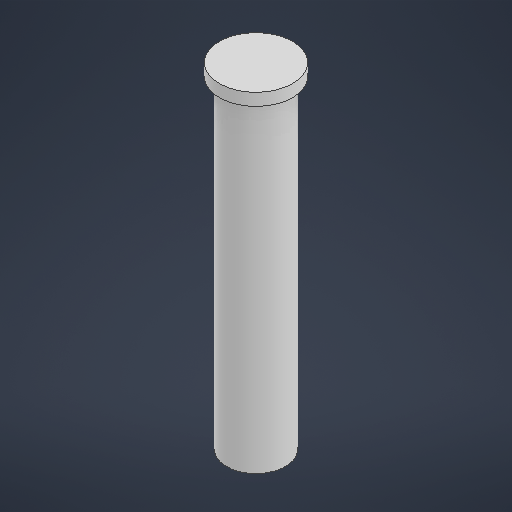
# Autodesk Inventor part: Press_Head
Saved by Autodesk Inventor 2026.1 (Build 301233020, 233B)
## iProperties
Created: 2025-09-29
Part Number: Press_Head
Material: Generic
Document SubType Name: Modeling
Designer: Gamec
Density: 1 g/cm^3
Appearance: Default
Author: Gamec
Autodesk Inventor part; units mm, degrees
ref_plane "YZ Plane" through (0, 0, 0) normal (1, 0, 0) x (0, 1, 0)
ref_plane "XZ Plane" through (0, 0, 0) normal (0, 1, 0) x (-1, 0, 0)
ref_plane "XY Plane" through (0, 0, 0) normal (0, 0, 1) x (1, 0, 0)
sketch "Sketch1" plane through (0, 0, 0) normal (0, 1, 0) x (-1, 0, 0)
  circle A0 centre (0, 0) radius 6.15
  dimension "d0" = 12.3
  constraints: 1 centre point, 1 coincident
  measures "d0" diameter of A0
extrude "Extrusion1" add sketch "Sketch1" along normal blind 69.85
sketch "Sketch2" plane through (0, 69.85, 0) normal (0, 1, 0) x (1, 0, 0)
  circle A0 centre (0, 0) radius 6.7945
  circle A1 centre (0, 0) radius 7.62
  dimension "d3" = 15.24
  constraints: 2 centre point, 2 coincident
  measures "d3" diameter of A1
extrude "Extrusion2" add sketch "Sketch2" against normal blind 2.54 contours A0 | A1
sketch "Sketch3" plane through (0, 0, 0) normal (0, -1, 0) x (1, 0, 0)
  circle A0 centre (0, 0) radius 3.9
  dimension "d6" = 7.8
  constraints: 1 centre point, 1 coincident
  measures "d6" diameter of A0
extrude "Extrusion3" cut sketch "Sketch3" against normal blind 50.8
body "Solid1"
